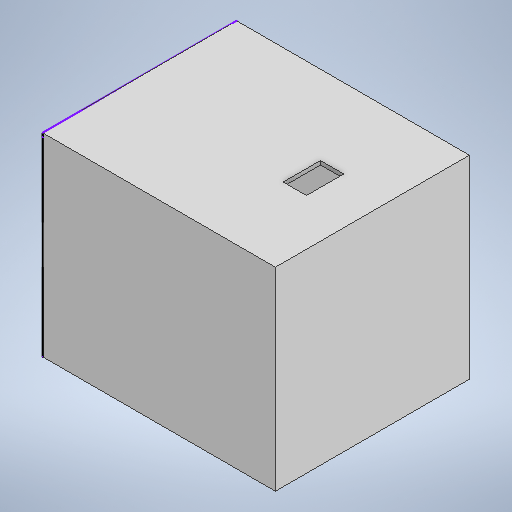
# Autodesk Inventor part: box-1
Saved by Autodesk Inventor 2025.2 (Build 292293000, 293)
## iProperties
Created: 2025-02-03
Part Number: box-1
Material: Generic
Document SubType Name: Modeling
Designer: sujay
Density: 1 g/cm^3
Appearance: Default
Author: sujay
Autodesk Inventor part; units mm, degrees
ref_plane "YZ Plane" through (0, 0, 0) normal (1, 0, 0) x (0, 1, 0)
ref_plane "XZ Plane" through (0, 0, 0) normal (0, 1, 0) x (-1, 0, 0)
ref_plane "XY Plane" through (0, 0, 0) normal (0, 0, 1) x (1, 0, 0)
sketch "Sketch1" plane through (0, 0, 0) normal (1, 0, 0) x (0, 1, 0)
  line L0 (0, 0) -> (127, 0)
  line L1 (127, 0) -> (127, -127)
  line L2 (127, -127) -> (0, -127)
  line L3 (0, -127) -> (0, 0)
  line L4 (127, -127) -> (124.46, -127)
  line L5 (124.46, -127) -> (124.46, -124.46)
  line L6 (124.46, -124.46) -> (127, -124.46)
  line L7 (127, -124.46) -> (127, -127)
  line L8 (127, 0) -> (124.46, 0)
  line L9 (124.46, 0) -> (124.46, -2.54)
  line L10 (124.46, -2.54) -> (127, -2.54)
  line L11 (127, -2.54) -> (127, 0)
  line L12 (124.46, -2.54) -> (2.54, -2.54)
  line L13 (2.54, -2.54) -> (2.54, -124.46)
  line L14 (2.54, -124.46) -> (124.46, -124.46)
  line L15 (124.46, -124.46) -> (124.46, -2.54)
  line L16 (124.46, -124.46) -> (122.682, -124.46)
  line L17 (124.46, -2.54) -> (68.58, -2.54)
  line L18 (124.46, -4.572) -> (124.46, -2.54)
  line L19 (0, 0) -> (50.8, 0)
  line L20 (0, -25.4) -> (0, 0)
  line L21 (127, 0) -> (76.2, 0)
  line L22 (127, -25.4) -> (127, 0)
  constraints: 46 end point, 8 parallel, 7 horizontal, 4 perpendicular, 1 point on line
extrude "Extrusion1" add sketch "Sketch1" along normal blind 152.4
extrude "Extrusion2" cut sketch "Sketch1" along normal blind 149.86 contours L15 L14 L13 L12
sketch "Sketch10" plane through (0, 2.54, -124.46) normal (0, 0, 1) x (1, 0, 0)
  line L0 (0, 0) -> (149.86, 0) projected
  line L1 (149.86, 0) -> (90.17, 0)
  line L2 (90.17, 0) -> (90.17, 2.032)
  line L3 (90.17, 2.032) -> (149.86, 2.032)
  line L4 (149.86, 2.032) -> (149.86, 0)
  line L5 (0, 0) -> (90.17, 2.032)
  point P0 (0, -2.54)
  dimension "d22" = 59.69
  dimension "d23" = 2.032
  constraints: 10 end point, 2 parallel, 1 horizontal, 1 perpendicular
  measures "d22" distance of L2.end L3.end
  measures "d23" distance of L1.end L2.end
extrude "Extrusion5" add sketch "Sketch10" along normal blind 121.92
sketch "Sketch11" plane through (0, 127, 0) normal (0, 1, 0) x (1, 0, 0)
  line L0 (0, 0) -> (152.4, 0) projected
  line L1 (152.4, 0) -> (121.92, 0)
  line L2 (121.92, 0) -> (121.92, 50.8)
  line L3 (121.92, 50.8) -> (152.4, 50.8)
  line L4 (152.4, 50.8) -> (152.4, 0)
  line L5 (152.4, 126.0289) -> (121.92, 126.0289)
  line L6 (121.92, 126.0289) -> (121.92, 75.2289)
  line L7 (121.92, 75.2289) -> (152.4, 75.2289)
  line L8 (152.4, 75.2289) -> (152.4, 126.0289)
  line L9 (121.92, 75.2289) -> (106.68, 75.2289)
  line L10 (106.68, 75.2289) -> (106.68, 50.8)
  line L11 (106.68, 50.8) -> (121.92, 50.8)
  line L12 (121.92, 50.8) -> (121.92, 75.2289)
  dimension "d30" = 30.48
  dimension "d31" = 50.8
  dimension "d32" = 30.48
  dimension "d33" = 50.8
  dimension "d34" = 15.24
  constraints: 24 end point, 6 parallel, 3 horizontal, 3 perpendicular, 1 point on line
  measures "d30" distance of L2.end L3.end
  measures "d31" distance of L1.end L2.end
  measures "d32" distance of L7.end L6.end
  measures "d33" distance of L6.end L5.end
  measures "d34" distance of L11.end L10.end
extrude "Extrusion6" cut sketch "Sketch11" against normal blind 2.54 contours L11 L10 L9 L12
body "Solid1"
